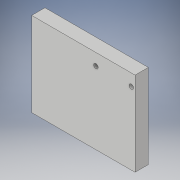
# Autodesk Inventor part: Small bumper Kermit
Saved by Autodesk Inventor 2018 (Build 220112000, 112)
## iProperties
Created: 2018-02-13
Part Number: Small bumper Kermit
Material: Generic
Document SubType Name: Modeling
Designer: kalra.rohan
Density: 1 g/cm^3
Appearance: Default
Author: kalra.rohan
Autodesk Inventor part; units mm, degrees
ref_plane "YZ Plane" through (0, 0, 0) normal (1, 0, 0) x (0, 1, 0)
ref_plane "XZ Plane" through (0, 0, 0) normal (0, 1, 0) x (-1, 0, 0)
ref_plane "XY Plane" through (0, 0, 0) normal (0, 0, 1) x (1, 0, 0)
sketch "Sketch1" plane through (0, 0, 0) normal (0, 0, 1) x (1, 0, 0)
  line L0 (0, 0) -> (177.8, 0)
  line L1 (177.8, 0) -> (177.8, -144.78)
  line L2 (177.8, -144.78) -> (0, -144.78)
  line L3 (0, -144.78) -> (0, 0)
  circle A0 centre (110.49, -20.32) radius 3.9179
  circle A1 centre (171.45, -20.32) radius 3.918
  dimension "d0" = 177.8
  dimension "d1" = 144.78
  dimension "d2" = 7.8359
  dimension "d3" = 124.46
  dimension "d4" = 110.49
  dimension "d5" = 7.8359
  dimension "d6" = 60.96
  constraints: 8 end point, 2 centre point, 2 parallel, 1 horizontal, 1 perpendicular
  measures "d0" distance between parallel lines of L1 L3
  measures "d1" distance between parallel lines of L2 L0
  measures "d2" diameter of A0
  measures "d3" distance from line of A0.centre L2
  measures "d4" distance from line of A0.centre L3
  measures "d5" diameter of A1
  measures "d6" distance of A1.centre A0.centre
extrude "Extrusion1" add sketch "Sketch1" against normal blind 22.86
body "Solid1"
